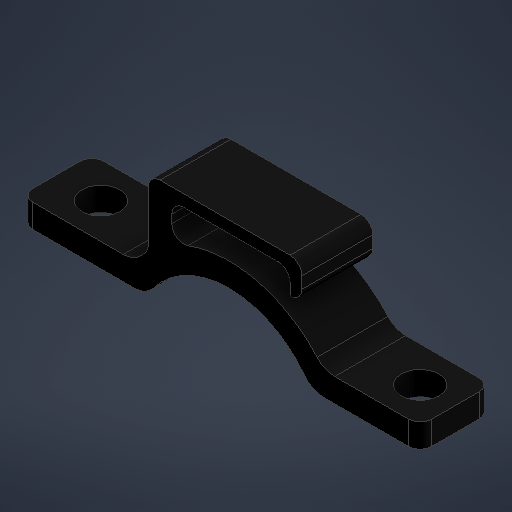
# Autodesk Inventor part: DribblerMotorKlemme
Saved by Autodesk Inventor 2025.2 (Build 292293000, 293)
## iProperties
Created: 2025-02-03
Part Number: DribblerMotorKlemme
Material: Generisch
Document SubType Name: Modeling
Designer: Faabs
Density: 1 g/cm^3
Appearance: Vorgabe
Author: Faabs
Autodesk Inventor part; units mm, degrees
ref_plane "YZ Plane" through (0, 0, 0) normal (1, 0, 0) x (0, 1, 0)
ref_plane "XZ Plane" through (0, 0, 0) normal (0, 1, 0) x (-1, 0, 0)
ref_plane "XY Plane" through (0, 0, 0) normal (0, 0, 1) x (1, 0, 0)
sketch "Skizze1" plane through (0, 0, 0) normal (0, 0, 1) x (1, 0, 0)
  line L0 (30, 3) -> (30, -3)
  line L1 (30, -3) -> (-3.765, -3)
  line L2 (-3.765, -3) -> (-3.765, 3)
  line L3 (-3.765, 3) -> (30, 3)
  circle A0 centre (0, 0) radius 1.6
  circle A1 centre (0, 0) radius 1.6
  circle A2 centre (27, 0) radius 1.6
  circle A3 centre (27, 0) radius 1.6
  line L4 (21.832, 1.0001) -> (21.832, -3)
  line L5 (21.832, -3) -> (5.832, -3)
  line L6 (5.832, -3) -> (5.832, 1.0001)
  line L7 (5.832, 1.0001) -> (21.832, 1.0001)
  dimension "d0" = 6
  constraints: 16 end point, 4 centre point, 4 parallel, 2 coincident, 2 perpendicular, 1 point on line
  measures "d0" distance of L1.end L2.end
extrude "Extrusion1" add sketch "Skizze1" along normal blind 7
sketch "Skizze2" plane through (-3.765, -3, 0) normal (0, -1, 0) x (1, 0, 0)
  line L0 (0, 0) -> (33.765, 0) projected
  line L1 (0, 0) -> (9.597, 0)
  line L2 (9.597, 0) -> (25.597, 0)
  line L3 (17.597, 0) -> (17.597, -4)
  circle A0 centre (17.597, -4) radius 8
  line L4 (0, 0) -> (0, 2)
  circle A1 centre (17.597, -4) radius 10
  line L5 (0, 2) -> (9.597, 2)
  line L6 (0, 0) -> (0, 7) projected
  line L7 (33.765, 0) -> (33.765, 2)
  line L8 (33.765, 0) -> (33.765, 7) projected
  line L9 (33.765, 2) -> (25.597, 2)
  line L10 (33.765, 7) -> (0, 7) projected
  line L11 (0, 7) -> (33.765, 7)
  line L12 (33.765, 7) -> (33.765, 0)
  line L13 (33.765, 0) -> (0, 0)
  line L14 (0, 0) -> (0, 7)
  point P0 (3.765, 0)
  point P1 (24.5252, 0)
  point P2 (10.6688, 0)
  point P3 (17.597, 7)
  point P4 (8.4318, 0)
  point P5 (26.7622, 0)
  dimension "d3" = 9.597
  dimension "d4" = 16
  dimension "d5" = 4
  dimension "d6" = 16
  dimension "d7" = 2
  dimension "d8" = 2
  dimension "d9" = 2
  constraints: 22 end point, 4 perpendicular, 3 point on line, 2 centre point, 2 parallel, 2 point on circle, 1 coincident, 1 horizontal, 1 midpoint, 1 vertical
  measures "d3" distance of L0.start L1.end
  measures "d4" distance of L1.end L2.end
  measures "d5" distance of L3.start L3.end
  measures "d6" diameter of A0
  measures "d7" distance of L0.start L4.end
  measures "d8" radial gap between concentric circles of A0 A1
  measures "d9" distance of L0.end L7.end
extrude "Extrusion2" cut sketch "Skizze2" against normal blind 7 contours L6 L10 L8 L9 A1 L5 | A0 L0 picked at (13.3479, 0.4966)
fillet "Rundung1" radius 2 4 edges at (5.832, 0, 2) (6.9038, 0, 0) (20.7602, 0, 0) (21.832, 0, 2)
fillet "Rundung2" radius 1 4 edges at (-3.765, -3, 1) (30, -3, 1) (30, 3, 1) (-3.765, 3, 1)
sketch "Skizze3" plane through (13.832, -3, -4) normal (0, -1, 0) x (1, 0, 0)
  line L0 (-13.832, 4) -> (-6.832, 4)
  line L1 (-15.432, 3) -> (-12.232, 3) projected
  line L2 (-6.832, 4) -> (-6.832, 13)
  line L3 (-6.832, 13) -> (6.168, 13)
  line L4 (6.168, 13) -> (6.168, 10)
  line L5 (6.168, 10) -> (5.168, 10)
  line L6 (5.168, 10) -> (5.168, 12)
  line L7 (5.168, 12) -> (-4.832, 12)
  line L8 (-4.832, 12) -> (-4.832, 8.7551)
  arc A0 (7.4536, 6.6667) -> (-7.4536, 6.6667) centre (0, 0) ccw projected
  arc A1 (7.4536, 6.6667) -> (-7.4536, 6.6667) centre (0, 0) ccw
  point P0 (-13.832, 4)
  point P1 (-12.232, 3)
  point P2 (-6.832, 7.3023)
  point P3 (9.1652, 4)
  point P4 (-9.1652, 4)
  dimension "d14" = 7
  dimension "d15" = 9
  dimension "d16" = 13
  dimension "d17" = 3
  dimension "d18" = 1
  dimension "d19" = 2
  dimension "d20" = 10
  constraints: 14 end point, 5 perpendicular, 3 point on circle, 2 vertical, 1 centre point, 1 concentric, 4 other
  measures "d14" distance of point (-13.832, 4) L2.start
  measures "d15" distance of L2.start L2.end
  measures "d16" distance of L2.end L3.end
  measures "d17" distance of L3.end L4.end
  measures "d18" distance of L4.end L5.end
  measures "d19" distance of L5.end L6.end
  measures "d20" distance of L6.end L7.end
extrude "Extrusion3" add sketch "Skizze3" against normal up to surface (6 mm away)
fillet "Rundung3" radius 1 7 edges at (20, 0, 6) (20, 0, 9) (7, 0, 9) (19, 0, 8) (9, 0, 8) (9, 0, 4.7551) (7, 0, 3.3023)
fillet "Rundung4" radius 0.2 2 edges at (19.0001, 0, 6) (19, 0, 6)
